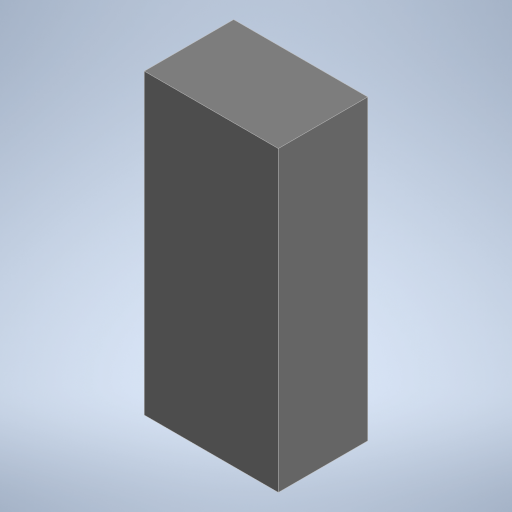
# Autodesk Inventor part: sponge
Saved by Autodesk Inventor 2024 (Build 280153000, 153)
## iProperties
Created: 2025-02-08
Part Number: sponge
Material: ゴム
Document SubType Name: Modeling
Designer: 1412z
Density: 0.93 g/cm^3
Appearance: 灰色
Author: 1412z
Autodesk Inventor part; units mm, degrees
ref_plane "YZ Plane" through (0, 0, 0) normal (1, 0, 0) x (0, 1, 0)
ref_plane "XZ Plane" through (0, 0, 0) normal (0, 1, 0) x (-1, 0, 0)
ref_plane "XY Plane" through (0, 0, 0) normal (0, 0, 1) x (1, 0, 0)
sketch "スケッチ1" plane through (0, 0, 0) normal (0, 0, 1) x (1, 0, 0)
  line L0 (-2.25, -5) -> (2.25, -5)
  line L1 (2.25, -5) -> (2.25, 5)
  line L2 (2.25, 5) -> (-2.25, 5)
  line L3 (-2.25, 5) -> (-2.25, -5)
  line L4 (-2.25, -5) -> (2.25, 5) construction
  line L5 (2.25, -5) -> (-2.25, 5) construction
  point P0 (0, 0)
  dimension "d0" = 4.5
  dimension "d1" = 10
  constraints: 12 end point, 2 midpoint, 2 parallel, 1 horizontal, 1 perpendicular
  measures "d0" distance of L2.end L1.end
  measures "d1" distance of L1.end L0.end
extrude "押し出し1" add sketch "スケッチ1" along normal blind 3
